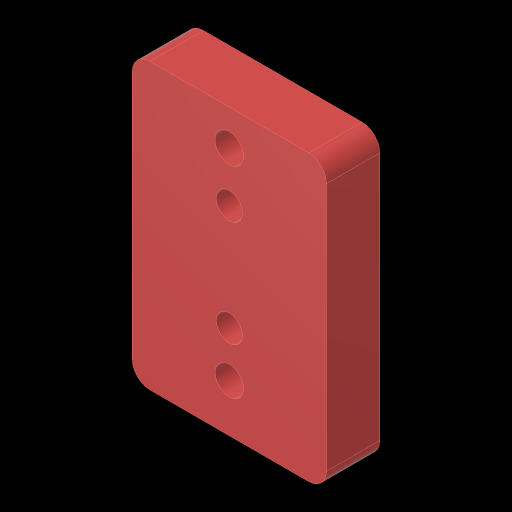
# Autodesk Inventor part: anderson battery connectorAnderson adapter
Saved by Autodesk Inventor 2023.3 (Build 273359000, 359)
## iProperties
Created: 2024-02-22
Part Number: anderson battery connectorAnderson adapter
Material: ABS Plastic
Document SubType Name: Modeling
Designer: slick
Density: 1.06 g/cm^3
Appearance: Smooth - Red
Author: slick
Autodesk Inventor part; units mm, degrees
ref_plane "YZ Plane" through (0, 0, 0) normal (1, 0, 0) x (0, 1, 0)
ref_plane "XZ Plane" through (0, 0, 0) normal (0, 1, 0) x (-1, 0, 0)
ref_plane "XY Plane" through (0, 0, 0) normal (0, 0, 1) x (1, 0, 0)
sketch "Sketch1" plane through (0, 0, 0) normal (0, 0, 1) x (1, 0, 0)
  line L0 (-17.3375, 25.4) -> (17.3375, 25.4)
  line L1 (17.3375, 25.4) -> (17.3375, -25.4)
  line L2 (17.3375, -25.4) -> (-17.3375, -25.4)
  line L3 (-17.3375, -25.4) -> (-17.3375, 25.4)
  line L4 (-17.3375, 25.4) -> (17.3375, -25.4) construction
  line L5 (17.3375, 25.4) -> (-17.3375, -25.4) construction
  line L6 (0, 19.05) -> (0, -16.871) construction
  line L7 (0, 10.16) -> (0, -8.756) construction
  point P0 (0, 0)
  point P1 (0, 0.702)
  point P2 (0, 25.4)
  point P3 (0, 1.0895)
  dimension "d0" = 34.675
  dimension "d1" = 50.8
  dimension "d3" = 18.916
  dimension "d4" = 15.24
  dimension "d23" = 35.921
  dimension "d26" = 6.35
  constraints: 16 end point, 5 midpoint, 2 parallel, 2 vertical alignment, 1 horizontal, 1 perpendicular, 1 point on line, 1 vertical
  measures "d0" distance of L0.start L0.end
  measures "d1" distance of L2.end L0.start
  measures "d3" distance of L7.end L7.start
  measures "d4" distance from line of L0 L7.start
  measures "d23" distance of L6.start L6.end
  measures "d26" distance of point (0, 25.4) L6.start
extrude "Extrusion1" add sketch "Sketch1" along normal blind 9.525
hole "Hole1" at (0, 19.05, 0) at (0, -16.871, 0) direction (0, 0, 1) diameter 5.1054 end through all counterbore diameter 9.525 counterbore depth 4.826 clearance for "Socket Head Cap Screw" size "#10" standard "Ansi Unified Screw Threads"
hole "Hole2" at (0, -8.756, 0) at (0, 10.16, 0) direction (0, 0, 1) diameter 4.7 end through all
fillet "Fillet1" radius 3.175 4 edges at (17.3375, 25.4, 4.7625) (-17.3375, 25.4, 4.7625) (-17.3375, -25.4, 4.7625) (17.3375, -25.4, 4.7625)
body "Solid1"
